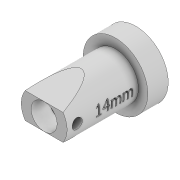
# Autodesk Inventor part: 200610 - 7-5mm lens adapter for half inch tube - MEMS side
Saved by Autodesk Inventor 2020.3 (Build 243373000, 373)
## iProperties
Created: 2020-06-10
Part Number: 200610 - 7-5mm lens adapter for half inch tube - MEMS side
Material: Generic
Document SubType Name: Modeling
Designer: Ralf
Density: 1 g/cm^3
Appearance: Default
Author: Ralf
Autodesk Inventor part; units mm, degrees
ref_plane "XZ Plane" through (0, 0, 0) normal (0, 1, 0) x (-1, 0, 0)
ref_plane "XY Plane" through (0, 0, 0) normal (0, 0, 1) x (1, 0, 0)
sketch "Sketch1" plane through (0, 0, 0) normal (0, 0, 1) x (1, 0, 0)
  circle A0 centre (0, 0) radius 6.35
  circle A1 centre (0, 0) radius 4
  dimension "d0" = 12.7
  dimension "d1" = 8
  constraints: 2 centre point, 2 coincident
  measures "d0" diameter of A0
  measures "d1" diameter of A1
extrude "Extrusion1" add sketch "Sketch1" along normal blind 4
sketch "Sketch2" plane through (0, 0, 4) normal (0, 0, 1) x (1, 0, 0)
  circle A0 centre (0, 0) radius 4.5
  dimension "d4" = 9
  constraints: 1 centre point, 1 coincident
  measures "d4" diameter of A0
extrude "Extrusion2" add sketch "Sketch2" along normal blind 14
sketch "Sketch3" plane through (0, 0, 18) normal (0, 0, 1) x (1, 0, 0)
  circle A0 centre (0, 0) radius 2.45
  dimension "d7" = 4.9
  constraints: 1 centre point, 1 coincident
  measures "d7" diameter of A0
extrude "Extrusion3" cut sketch "Sketch3" against normal blind 30
sketch "Sketch4" plane through (0, 0, 0) normal (1, 0, 0) x (0, 1, 0)
  line L0 (4.5, 18) -> (-4.5, 18) projected
  line L1 (0, 18) -> (2.55, 18)
  line L2 (2.55, 18) -> (4.5, 10.7225)
  line L3 (4.5, 4) -> (4.5, 18) projected
  line L4 (4.5, 10.7225) -> (4.5, 18)
  line L5 (2.55, 18) -> (4.5, 10.7225)
  line L6 (0, 18) -> (-2.55, 18)
  line L7 (-2.55, 18) -> (-4.5, 10.7225)
  line L8 (-4.5, 4) -> (-4.5, 18) projected
  line L9 (-4.5, 10.7225) -> (-4.5, 18)
  line L10 (-2.55, 18) -> (-4.5, 18)
  point P0 (0, 0)
  dimension "d10" = 2.55
  dimension "d11" = 105
  dimension "d14" = 2.55
  dimension "d15" = 105
  constraints: 16 end point, 6 point on line, 2 collinear, 1 midpoint, 1 perpendicular
  measures "d10" distance of L1.start L1.end
  measures "d11" angle of L1 L2
  measures "d14" distance of L1.start L6.end
  measures "d15" angle of L7 L6
extrude "Extrusion4" cut sketch "Sketch4" along normal mid plane 10
ref_plane "Work Plane1" through (4.5, 0, 0) normal (1, 0, 0) x (0, 1, 0)
sketch "Sketch6" plane through (4.5, 0, 0) normal (1, 0, 0) x (0, 1, 0)
  line L0 (1.1727, 12.5271) -> (1.1727, 7.4672) construction
  line L1 (1.1727, 7.4672) -> (0.1306, 7.4672) construction
  line L2 (0.1306, 7.4672) -> (0.1306, 12.5271) construction
  line L3 (0.1306, 12.5271) -> (1.1727, 12.5271) construction
  line L4 (-0.8338, 11.2483) -> (-0.8338, 12.224)
  line L5 (-0.8338, 12.224) -> (-0.6296, 12.224)
  line L6 (-0.6296, 12.224) -> (-0.6296, 11.861)
  line L7 (-0.6296, 11.861) -> (0.7108, 11.861)
  line L8 (0.7108, 11.861) -> (0.7108, 12.224)
  line L9 (0.7108, 12.224) -> (0.8939, 12.224)
  spline S0 degree 2 poles (0.8939, 12.224) (0.8939, 12.0182) (1.0106, 11.8237) (1.1727, 11.8107) knots 0 0 0 1 2 2 2
  line L10 (1.1727, 11.8107) -> (1.1727, 11.6033)
  line L11 (1.1727, 11.6033) -> (-0.6296, 11.6033)
  line L12 (-0.6296, 11.6033) -> (-0.6296, 11.2483)
  line L13 (-0.6296, 11.2483) -> (-0.8338, 11.2483)
  line L14 (-0.1466, 9.5936) -> (-0.1466, 9.8318)
  line L15 (-0.1466, 9.8318) -> (-0.8338, 9.8318)
  line L16 (-0.8338, 9.8318) -> (-0.8338, 10.0895)
  line L17 (-0.8338, 10.0895) -> (-0.1466, 10.0895)
  line L18 (-0.1466, 10.0895) -> (-0.1466, 10.9728)
  line L19 (-0.1466, 10.9728) -> (0.1354, 10.9728)
  line L20 (0.1354, 10.9728) -> (1.1662, 10.0782)
  line L21 (1.1662, 10.0782) -> (1.1662, 9.8318)
  line L22 (1.1662, 9.8318) -> (0.069, 9.8318)
  line L23 (0.069, 9.8318) -> (0.069, 9.5936)
  line L24 (0.069, 9.5936) -> (-0.1466, 9.5936)
  line L25 (0.069, 10.0895) -> (0.8502, 10.0895)
  line L26 (0.8502, 10.0895) -> (0.069, 10.7621)
  line L27 (0.069, 10.7621) -> (0.069, 10.0895)
  line L28 (-0.8338, 7.6406) -> (0.0349, 7.6406)
  spline S1 degree 2 poles (0.0349, 7.6406) (0.1387, 7.6406) (0.3153, 7.6568) (0.364, 7.6827) knots 0 0 0 1 2 2 2
  spline S2 degree 2 poles (0.364, 7.6827) (0.4174, 7.7086) (0.4693, 7.8075) (0.4693, 7.8934) knots 0 0 0 1 2 2 2
  spline S3 degree 2 poles (0.4693, 7.8934) (0.4693, 7.9712) (0.3737, 8.1495) (0.2829, 8.2435) knots 0 0 0 1 2 2 2
  spline S4 degree 2 poles (0.2829, 8.2435) (0.2602, 8.2419) (0.197, 8.2386) (0.1549, 8.2386) knots 0 0 0 1 2 2 2
  line L29 (0.1549, 8.2386) -> (-0.8338, 8.2386)
  line L30 (-0.8338, 8.2386) -> (-0.8338, 8.4915)
  line L31 (-0.8338, 8.4915) -> (0.0349, 8.4915)
  spline S5 degree 2 poles (0.0349, 8.4915) (0.1387, 8.4915) (0.3153, 8.5077) (0.364, 8.5336) knots 0 0 0 1 2 2 2
  spline S6 degree 2 poles (0.364, 8.5336) (0.4174, 8.5595) (0.4693, 8.6584) (0.4693, 8.7443) knots 0 0 0 1 2 2 2
  spline S7 degree 2 poles (0.4693, 8.7443) (0.4693, 8.8253) (0.3672, 9.0052) (0.2878, 9.0895) knots 0 0 0 1 2 2 2
  line L32 (0.2878, 9.0895) -> (-0.8338, 9.0895)
  line L33 (-0.8338, 9.0895) -> (-0.8338, 9.3424)
  line L34 (-0.8338, 9.3424) -> (0.667, 9.3424)
  line L35 (0.667, 9.3424) -> (0.667, 9.0895)
  line L36 (0.667, 9.0895) -> (0.5017, 9.0895)
  spline S8 degree 2 poles (0.5017, 9.0895) (0.6006, 8.9907) (0.7092, 8.7962) (0.7092, 8.6795) knots 0 0 0 1 2 2 2
  spline S9 degree 2 poles (0.7092, 8.6795) (0.7092, 8.5466) (0.5876, 8.3407) (0.4499, 8.2872) knots 0 0 0 1 2 2 2
  spline S10 degree 2 poles (0.4499, 8.2872) (0.5779, 8.1722) (0.7092, 7.955) (0.7092, 7.8286) knots 0 0 0 1 2 2 2
  spline S11 degree 2 poles (0.7092, 7.8286) (0.7092, 7.7313) (0.6492, 7.5725) (0.5811, 7.5142) knots 0 0 0 1 2 2 2
  spline S12 degree 2 poles (0.5811, 7.5142) (0.5131, 7.4542) (0.3088, 7.3877) (0.1549, 7.3877) knots 0 0 0 1 2 2 2
  line L37 (0.1549, 7.3877) -> (-0.8338, 7.3877)
  line L38 (-0.8338, 7.3877) -> (-0.8338, 7.6406)
  line L39 (-0.8338, 5.331) -> (0.0349, 5.331)
  spline S13 degree 2 poles (0.0349, 5.331) (0.1387, 5.331) (0.3153, 5.3472) (0.364, 5.3731) knots 0 0 0 1 2 2 2
  spline S14 degree 2 poles (0.364, 5.3731) (0.4174, 5.3991) (0.4693, 5.4979) (0.4693, 5.5838) knots 0 0 0 1 2 2 2
  spline S15 degree 2 poles (0.4693, 5.5838) (0.4693, 5.6616) (0.3737, 5.8399) (0.2829, 5.9339) knots 0 0 0 1 2 2 2
  spline S16 degree 2 poles (0.2829, 5.9339) (0.2602, 5.9323) (0.197, 5.9291) (0.1549, 5.9291) knots 0 0 0 1 2 2 2
  line L40 (0.1549, 5.9291) -> (-0.8338, 5.9291)
  line L41 (-0.8338, 5.9291) -> (-0.8338, 6.1819)
  line L42 (-0.8338, 6.1819) -> (0.0349, 6.1819)
  spline S17 degree 2 poles (0.0349, 6.1819) (0.1387, 6.1819) (0.3153, 6.1981) (0.364, 6.224) knots 0 0 0 1 2 2 2
  spline S18 degree 2 poles (0.364, 6.224) (0.4174, 6.25) (0.4693, 6.3488) (0.4693, 6.4347) knots 0 0 0 1 2 2 2
  spline S19 degree 2 poles (0.4693, 6.4347) (0.4693, 6.5158) (0.3672, 6.6957) (0.2878, 6.78) knots 0 0 0 1 2 2 2
  line L43 (0.2878, 6.78) -> (-0.8338, 6.78)
  line L44 (-0.8338, 6.78) -> (-0.8338, 7.0328)
  line L45 (-0.8338, 7.0328) -> (0.667, 7.0328)
  line L46 (0.667, 7.0328) -> (0.667, 6.78)
  line L47 (0.667, 6.78) -> (0.5017, 6.78)
  spline S20 degree 2 poles (0.5017, 6.78) (0.6006, 6.6811) (0.7092, 6.4866) (0.7092, 6.3699) knots 0 0 0 1 2 2 2
  spline S21 degree 2 poles (0.7092, 6.3699) (0.7092, 6.237) (0.5876, 6.0312) (0.4499, 5.9777) knots 0 0 0 1 2 2 2
  spline S22 degree 2 poles (0.4499, 5.9777) (0.5779, 5.8626) (0.7092, 5.6454) (0.7092, 5.519) knots 0 0 0 1 2 2 2
  spline S23 degree 2 poles (0.7092, 5.519) (0.7092, 5.4218) (0.6492, 5.2629) (0.5811, 5.2046) knots 0 0 0 1 2 2 2
  spline S24 degree 2 poles (0.5811, 5.2046) (0.5131, 5.1446) (0.3088, 5.0782) (0.1549, 5.0782) knots 0 0 0 1 2 2 2
  line L48 (0.1549, 5.0782) -> (-0.8338, 5.0782)
  line L49 (-0.8338, 5.0782) -> (-0.8338, 5.331)
  point P0 (0, 0)
  constraints: 2 other
extrude "Extrusion5" cut sketch "Sketch6" against normal blind 0.5
sketch "Sketch8" plane through (0, 0, 18) normal (0, 0, 1) x (1, 0, 0)
  circle A0 centre (0, 0) radius 2.55
  dimension "d21" = 5.1
  constraints: 1 centre point, 1 coincident
  measures "d21" diameter of A0
extrude "Extrusion6" cut sketch "Sketch8" against normal blind 3.5
sketch "Sketch7" plane through (4.5, 0, 0) normal (1, 0, 0) x (0, 1, 0)
  circle A0 centre (0, 16) radius 1
  line L0 (2.55, 18) -> (-2.55, 18) projected
  point P0 (0, 0)
  dimension "d19" = 2
  dimension "d20" = 2
  constraints: 1 centre point
  measures "d19" diameter of A0
  measures "d20" distance from line of A0.centre L0
extrude "Extrusion7" cut sketch "Sketch7" against normal blind 5
body "Solid1"
